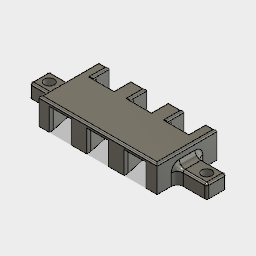
DC-Jack-Hookup-Mount (Autodesk Fusion 360 design; units mm, degrees)
Autodesk Fusion 360 part; units mm, degrees
sketch "Sketch3" plane through (0, 0, 0) normal (1, 0, 0) x (0, 0, -1)
  line L0 (-4.5, 11.51) -> (-16.25, 11.51)
  line L1 (-16.25, 11.51) -> (-26.45, 11.21)
  line L2 (-26.45, 11.21) -> (-26.45, 0)
  line L3 (-26.45, 0) -> (0, 0)
  line L4 (-4.5, 11.51) -> (-4.5, 0.01)
  line L5 (-4.5, 0.01) -> (0, 0.01)
  line L6 (0, 0.01) -> (0, 0)
  line L7 (2, 0) -> (-28.45, 0)
  line L8 (-28.45, 0) -> (-28.45, 13.51)
  line L9 (-28.45, 13.51) -> (2, 13.51)
  line L10 (2, 13.51) -> (2, 0)
  dimension "d19" = 11.75
  dimension "d21" = 0.01
  dimension "d22" = 4.5
  dimension "d24" = 11.5
  dimension "d63" = 2
  dimension "d64" = 2
  dimension "d65" = 2
  dimension "d68" = 0.3
  dimension "d69" = 10.2
  constraint perpendicular L0 L2
  constraint perpendicular L0 L4
  constraint perpendicular L4 L5
  constraint perpendicular L5 L6
  constraint horizontal L7
  constraint vertical L8
  constraint horizontal L9
  constraint vertical L10
  measures "d63" distance of L2 L8
  measures "d64" distance of L6 L10
  measures "d65" distance of L0 L9
extrude "Extrude3" add sketch "Sketch3" along normal blind 60 contours L0 L1 L2 L4 L5 L6 L7 L8 L9 L10
sketch "Sketch12" plane through (0, 13.51, 0) normal (0, 1, 0) x (-1, 0, 0)
  line L0 (0, -2) -> (0, 28.45)
  line L1 (0, 28.45) -> (-60, 28.45)
  line L2 (-60, 28.45) -> (-60, -2)
  line L3 (-60, -2) -> (0, -2)
  line L4 (-3, 4.5) -> (-3, 16.25)
  line L5 (0, 16.25) -> (0, 4.5)
  line L6 (0, 26.45) -> (-60, 26.45)
  line L7 (-3, 16.25) -> (-5.25, 26.45)
  line L8 (0, 4.5) -> (-60, 4.5) construction
  line L9 (-18.5, 16.25) -> (-18.5, 4.5)
  line L10 (-18.5, 16.25) -> (0, 16.25) construction
  line L11 (-18.5, 16.25) -> (-16.25, 26.45)
  line L12 (-3, 4.5) -> (-5.25, 4.5)
  line L13 (-3, 4.5) -> (-0.198, 4.5) construction
  line L14 (-5.25, 4.5) -> (-5.25, -2)
  line L15 (-5.25, -2) -> (-16.25, -2)
  line L16 (-16.25, -2) -> (-16.25, 4.5)
  line L17 (-16.25, 4.5) -> (-18.5, 4.5)
  line L18 (-16.25, 4.5) -> (-18.5, 4.5)
  line L19 (-22, 16.25) -> (-24.25, 26.45)
  line L20 (-22, 4.5) -> (-24.25, 4.5)
  line L21 (-24.25, 4.5) -> (-24.25, -2)
  line L22 (-22, 4.5) -> (-22, 16.25)
  line L23 (-24.25, -2) -> (-35.25, -2)
  line L24 (-37.5, 16.25) -> (-35.25, 26.45)
  line L25 (-35.25, 4.5) -> (-37.5, 4.5)
  line L26 (-35.25, -2) -> (-35.25, 4.5)
  line L27 (-35.25, 4.5) -> (-37.5, 4.5)
  line L28 (-37.5, 16.25) -> (-37.5, 4.5)
  line L29 (-41, 16.25) -> (-43.25, 26.45)
  line L30 (-41, 4.5) -> (-43.25, 4.5)
  line L31 (-43.25, 4.5) -> (-43.25, -2)
  line L32 (-41, 4.5) -> (-41, 16.25)
  line L33 (-43.25, -2) -> (-54.25, -2)
  line L34 (-56.5, 16.25) -> (-54.25, 26.45)
  line L35 (-54.25, 4.5) -> (-56.5, 4.5)
  line L36 (-54.25, -2) -> (-54.25, 4.5)
  line L37 (-54.25, 4.5) -> (-56.5, 4.5)
  line L38 (-56.5, 16.25) -> (-56.5, 4.5)
  dimension "d66" = 3
  dimension "d67" = 2.25
  dimension "d71" = 11.75
  dimension "d72" = 15.5
  dimension "d73" = 2.25
  dimension "d74" = 10.5
  dimension "d75" = 2.25
  dimension "d79" = 2.25
  dimension "d89" = -38
  dimension "d90" = 0
  constraint vertical L4
  constraint horizontal L10
  constraint coincident L6
  constraint coincident L8
  constraint perpendicular L4 L12
  constraint horizontal L13
  constraint perpendicular L3 L14
  constraint perpendicular L14 L15
  constraint vertical L16
  constraint collinear L3 L15
  constraint perpendicular L5 L10
extrude "Extrude15" add sketch "Sketch12" against normal blind 13.51 contours L0 L3 L4 L5 L6 L7 L12 L14 | L3 L6 L9 L11 L16 L17 L18 L19 L20 L21 L22 | L3 L6 L24 L25 L26 L27 L28 L29 L30 L31 L32 | L2 L3 L6 L34 L35 L36 L37 L38
sketch "Sketch13" plane through (0, 0, -2) normal (0, 0, -1) x (-1, 0, 0)
  line L0 (0, 13.51) -> (-60, 13.51)
  line L1 (-60, 13.51) -> (-60, 0)
  line L2 (-60, 0) -> (0, 0)
  line L3 (0, 0) -> (0, 13.51)
  line L4 (-5.25, 13.51) -> (-16.25, 13.51)
  line L5 (-16.25, 13.51) -> (-5.25, 13.51)
  line L6 (-5.25, 13.51) -> (-5.25, 0)
  line L7 (-5.25, 0) -> (-16.25, 0)
  line L8 (-16.25, 0) -> (-16.25, 13.51)
  line L9 (-54.25, 13.51) -> (-43.25, 13.51)
  line L10 (-43.25, 13.51) -> (-43.25, 0)
  line L11 (-43.25, 0) -> (-54.25, 0)
  line L12 (-54.25, 0) -> (-54.25, 13.51)
  line L13 (-35.25, 13.51) -> (-24.25, 13.51)
  line L14 (-24.25, 13.51) -> (-24.25, 0)
  line L15 (-24.25, 0) -> (-35.25, 0)
  line L16 (-35.25, 0) -> (-35.25, 13.51)
  constraint perpendicular L5 L6
  constraint parallel L5 L7
  constraint parallel L6 L8
  constraint parallel L4 L5
  constraint perpendicular L9 L10
  constraint parallel L9 L11
  constraint parallel L10 L12
  constraint parallel L0 L9
  constraint perpendicular L13 L14
  constraint parallel L13 L15
  constraint parallel L14 L16
  constraint perpendicular L12 L13
  constraint collinear L2 L7
extrude "Extrude13" cut sketch "Sketch13" against normal blind 8.5 contours L0 L2 L4 L5 L6 L7 L8 | L0 L2 L13 L14 L15 L16 | L0 L2 L9 L10 L11 L12
sketch "Sketch14" plane through (0, 0, 28.45) normal (0, 0, 1) x (1, 0, 0)
  line L0 (0, 13.51) -> (0, 0)
  line L1 (0, 0) -> (60, 0)
  line L2 (60, 0) -> (60, 13.51)
  line L3 (60, 13.51) -> (0, 13.51)
  line L4 (5.25, -0.0093) -> (5.25, 13.51) construction
  line L5 (16.25, 13.51) -> (16.25, 0) construction
  line L6 (5.25, 11.51) -> (16.25, 11.51)
  line L7 (16.25, 11.51) -> (16.25, 0)
  line L8 (16.25, 0) -> (5.25, 0)
  line L9 (5.25, 0) -> (5.25, 11.51)
  line L10 (24.25, 13.51) -> (24.25, 0) construction
  line L11 (35.25, 13.51) -> (35.25, 0) construction
  line L12 (43.25, 13.51) -> (43.25, 0) construction
  line L13 (54.25, 13.51) -> (54.25, 0) construction
  line L14 (24.25, 11.51) -> (35.25, 11.51)
  line L15 (35.25, 11.51) -> (35.25, 0)
  line L16 (35.25, 0) -> (24.25, 0)
  line L17 (24.25, 0) -> (24.25, 11.51)
  line L18 (43.25, 11.51) -> (54.25, 11.51)
  line L19 (54.25, 11.51) -> (54.25, 0)
  line L20 (54.25, 0) -> (43.25, 0)
  line L21 (43.25, 0) -> (43.25, 11.51)
  dimension "d84" = 2
  constraint vertical L4
  constraint coincident L1
  constraint perpendicular L1 L5
  constraint perpendicular L6 L7
  constraint parallel L6 L8
  constraint parallel L7 L9
  constraint coincident L5
  constraint coincident L4
  constraint perpendicular L1 L10
  constraint perpendicular L1 L11
  constraint perpendicular L1 L12
  constraint perpendicular L1 L13
  constraint horizontal L14
  constraint vertical L15
  constraint horizontal L16
  constraint vertical L17
  constraint horizontal L18
  constraint vertical L19
  constraint vertical L21
  constraint collinear L6 L18
  constraint coincident L10
  constraint collinear L6 L14
  measures "d84" distance of L3 L6
extrude "Extrude14" cut sketch "Sketch14" against normal blind 2 contours L1 L6 L7 L8 L9 | L1 L18 L19 L20 L21 | L1 L14 L15 L16 L17
sketch "Sketch5" plane through (0, 0, 0) normal (-1, 0, 0) x (0, 0, 1)
  line L0 (8.2, 0) -> (18.2, 0)
  line L1 (18.2, 0) -> (18.2, 7)
  line L2 (18.2, 7) -> (8.2, 7)
  line L3 (8.2, 7) -> (8.2, 0)
  line L4 (26.45, 0) -> (28.45, 0)
  line L5 (28.45, 0) -> (28.45, 13.51)
  line L6 (28.45, 13.51) -> (-2, 13.51)
  line L7 (-2, 13.51) -> (-2, 0)
  line L8 (4.5, 0.01) -> (4.5, 11.51)
  line L9 (4.5, 11.51) -> (16.25, 11.51)
  line L10 (16.25, 11.51) -> (26.45, 11.21)
  line L11 (26.45, 11.21) -> (26.45, 0)
  line L12 (-2, 0) -> (0, 0)
  line L13 (0, 0) -> (0, 0.01)
  line L14 (0, 0.01) -> (4.5, 0.01)
  dimension "d40" = 10
  dimension "d55" = 7
  constraint horizontal L0
  constraint vertical L1
  constraint horizontal L2
  constraint vertical L3
  constraint collinear L0 L4
extrude "Extrude5" add sketch "Sketch5" along normal blind 15 contours L0 L1 L2 L3
sketch "Sketch6" plane through (0, 7, 0) normal (0, 1, 0) x (-1, 0, 0)
  line L0 (0, 18.2) -> (0, 8.2)
  line L1 (0, 8.2) -> (15, 8.2)
  line L2 (15, 8.2) -> (15, 18.2)
  line L3 (15, 18.2) -> (0, 18.2)
  line L4 (15, 13.2) -> (0, 13.2) construction
  circle A0 centre (10, 13.2) radius 2.55
  dimension "d45" = 5.1
  dimension "d62" = 10
  constraint midpoint L2
  constraint midpoint L0
  constraint coincident L4
  measures "d45" diameter of A0
extrude "Extrude6" cut sketch "Sketch6" against normal blind 12 contours A0
sketch "Sketch10" plane through (60, 0, 0) normal (1, 0, 0) x (0, 0, -1)
  line L0 (-18.2, 7) -> (-8.2, 7)
  line L1 (-18.2, 7) -> (-8.2, 7)
  line L2 (-8.2, 7) -> (-8.2, 0)
  line L3 (-8.2, 0) -> (-18.2, 0)
  line L4 (-18.2, 0) -> (-18.2, 7)
  line L5 (0, 0) -> (2, 0)
  line L6 (2, 0) -> (2, 13.51)
  line L7 (2, 13.51) -> (-28.45, 13.51)
  line L8 (-28.45, 13.51) -> (-28.45, 0)
  line L9 (-4.5, 11.51) -> (-4.5, 0.01)
  line L10 (-4.5, 0.01) -> (0, 0.01)
  line L11 (0, 0.01) -> (0, 0)
  line L12 (-28.45, 0) -> (-26.45, 0)
  line L13 (-26.45, 0) -> (-26.45, 11.21)
  line L14 (-26.45, 11.21) -> (-16.25, 11.51)
  line L15 (-16.25, 11.51) -> (-4.5, 11.51)
  constraint perpendicular L1 L2
  constraint parallel L1 L3
  constraint parallel L2 L4
  constraint parallel L0 L1
extrude "Extrude10" add sketch "Sketch10" along normal blind 15 contours L0 L1 L2 L3 L4
sketch "Sketch11" plane through (0, 7, 0) normal (0, 1, 0) x (-1, 0, 0)
  line L0 (-60, 8.2) -> (-60, 18.2)
  line L1 (-60, 18.2) -> (-75, 18.2)
  line L2 (-75, 18.2) -> (-75, 8.2)
  line L3 (-75, 8.2) -> (-60, 8.2)
  line L4 (-60, 13.2) -> (-75, 13.2) construction
  circle A0 centre (-70, 13.2) radius 2.55
  dimension "d58" = 5.1
  dimension "d61" = 10
  constraint midpoint L0
  constraint midpoint L2
  constraint coincident L4
  measures "d58" diameter of A0
extrude "Extrude11" cut sketch "Sketch11" against normal blind 7 contours A0
fillet "Fillet1" radius 1 16 edges at (60, 13.51, 13.225) (30, 13.51, 28.45) (0, 13.51, 13.225) (10.75, 13.51, 6.5) (16.25, 13.51, 2.25) (20.25, 13.51, -2) (24.25, 13.51, 2.25) (29.75, 13.51, 6.5) (35.25, 13.51, 2.25) (39.25, 13.51, -2) (43.25, 13.51, 2.25) (48.75, 13.51, 6.5) (54.25, 13.51, 2.25) (57.125, 13.51, -2) (5.25, 13.51, 2.25) (2.625, 13.51, -2)
fillet "Fillet2" radius 1 10 edges at (-7.5, 7, 8.2) (-7.5, 7, 18.2) (-15, 7, 13.2) (75, 7, 13.2) (67.5, 7, 8.2) (67.5, 7, 18.2) (75, 3.5, 18.2) (75, 3.5, 8.2) (-15, 3.5, 8.2) (-15, 3.5, 18.2)
fillet "Fillet3" radius 3 10 edges at (0, 3, 8.2) (0, 6.7071, 8.4929) (0, 7, 13.2) (0, 6.7071, 17.9071) (0, 3, 18.2) (60, 3, 18.2) (60, 6.7071, 17.9071) (60, 7, 13.2) (60, 6.7071, 8.4929) (60, 3, 8.2)
equation "d67 = 3 mm - 0.75 mm"
equation "d69 = 10 mm + 0.2 mm"
equation "d72 = 15 mm + 0.5 mm"
equation "d73 = d67"
equation "d75 = 2.5 mm - 0.25 mm"
equation "d79 = d75"
